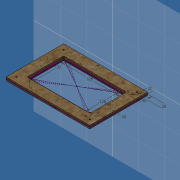
# Autodesk Inventor part: Flachfilter_Rahmen
Saved by Autodesk Inventor 2019 (Build 230136000, 136)
## iProperties
Created: 2020-08-04
Part Number: Flachfilter_Rahmen
Material: Generisch
Document SubType Name: Modeling
Designer: Stefan
Mass: 458.465 g
Surface Area: 1020.14 cm^2
Volume: 458.465 cm^3
Density: 1 g/cm^3
Appearance: Spanplatte
Author: Stefan
Autodesk Inventor part; units mm, degrees
ref_plane "YZ Plane" through (0, 0, 0) normal (1, 0, 0) x (0, 1, 0)
ref_plane "XZ Plane" through (0, 0, 0) normal (0, 1, 0) x (-1, 0, 0)
ref_plane "XY Plane" through (0, 0, 0) normal (0, 0, 1) x (1, 0, 0)
sketch "Skizze1" plane through (0, 0, 0) normal (0, 1, 0) x (-1, 0, 0)
  arc A0 (-116, -64) -> (-114, -66) centre (-114, -64) ccw
  arc A1 (-114, -62) -> (-112, -64) centre (-112, -62) ccw
  line L0 (-114, -62) -> (-114, 62)
  line L1 (-116, 64) -> (-116, -64)
  line L2 (-120, -65) -> (-120, 65)
  line L3 (112, -64) -> (-112, -64)
  line L4 (-114, -66) -> (114, -66)
  line L5 (115, -70) -> (-115, -70)
  line L6 (-112, 64) -> (112, 64)
  line L7 (114, 64) -> (-114, -64) construction
  line L8 (114, 66) -> (-114, 66)
  line L9 (-116, 66) -> (116, -66) construction
  line L10 (-116, -66) -> (116, 66) construction
  line L11 (-115, 70) -> (115, 70)
  line L12 (120, 70) -> (-120, -70) construction
  line L13 (120, -70) -> (-120, 70) construction
  line L14 (114, -64) -> (-114, 64) construction
  line L15 (120, 65) -> (120, -65)
  arc A2 (-120, -65) -> (-115, -70) centre (-115, -65) ccw
  arc A3 (-112, 64) -> (-114, 62) centre (-112, 62) ccw
  arc A4 (-115, 70) -> (-120, 65) centre (-115, 65) ccw
  arc A5 (-114, 66) -> (-116, 64) centre (-114, 64) ccw
  arc A6 (120, 65) -> (115, 70) centre (115, 65) ccw
  arc A7 (115, -70) -> (120, -65) centre (115, -65) ccw
  line L16 (116, -64) -> (116, 64)
  arc A8 (114, -66) -> (116, -64) centre (114, -64) ccw
  arc A9 (112, -64) -> (114, -62) centre (112, -62) ccw
  line L17 (114, 62) -> (114, -62)
  arc A10 (114, 62) -> (112, 64) centre (112, 62) ccw
  arc A11 (116, 64) -> (114, 66) centre (114, 64) ccw
  line L18 (-160, -110) -> (160, -110)
  line L19 (160, -110) -> (160, 110)
  line L20 (160, 110) -> (-160, 110)
  line L21 (-160, 110) -> (-160, -110)
  line L22 (-160, -110) -> (160, 110) construction
  line L23 (160, -110) -> (-160, 110) construction
  circle A12 centre (-140, -90) radius 2.75
  line L24 (140, 90) -> (-140, 90)
  line L25 (-140, 90) -> (-140, -90)
  line L26 (-140, -90) -> (140, -90)
  line L27 (140, -90) -> (140, 90)
  line L28 (140, 90) -> (-140, -90) construction
  line L29 (-140, 90) -> (140, -90) construction
  circle A13 centre (140, -90) radius 2.75
  circle A14 centre (140, 90) radius 2.75
  circle A15 centre (-140, 90) radius 2.75
  point P0 (0, 0)
  point P1 (0, 0)
  point P2 (0, 0)
  point P3 (0, 0)
  point P4 (0, 0)
  point P5 (0, 0)
  point P6 (0, 0)
  dimension "d0" = 140
  dimension "d1" = 240
  dimension "d2" = 5
  dimension "d3" = 232
  dimension "d4" = 132
  dimension "d5" = 2
  dimension "d6" = 128
  dimension "d7" = 228
  dimension "d8" = 2
  dimension "d19" = 40
  dimension "d20" = 40
  dimension "d21" = 5.5
  dimension "d23" = 20
  dimension "d24" = 20
  constraints: 60 end point, 24 point on circle, 24 point on line, 24 tangent, 16 centre point, 15 midpoint, 12 equal radius, 12 parallel, 5 coincident, 5 perpendicular, 3 horizontal
  measures "d0" distance of L12.end L13.end
  measures "d1" distance of L13.start L12.end
  measures "d2" radius of A6
  measures "d3" distance of L10.start L9.end
  measures "d4" distance of L9.end L10.end
  measures "d5" radius of A8
  measures "d6" distance of L7.end L14.end
  measures "d7" distance of L14.start L7.end
  measures "d8" radius of A9
  measures "d19" distance between parallel lines of L5 L18
  measures "d20" distance between parallel lines of L2 L21
  measures "d21" diameter of A12
  measures "d23" distance between parallel lines of L18 L26
  measures "d24" distance between parallel lines of L25 L21
extrude "Extrusion1" add sketch "Skizze1" along normal blind 6 contours L21 L20 L19 L18 | L26 L25 A12 | A12 L25 L26 | A12 L25 A15 L24 A14 L27 A13 L26 | A13 L27 L26 | L26 L27 A13 | A15 L24 L25 | L25 L24 A15 | A14 L24 L27 | L27 L24 A14
extrude "Extrusion2" add sketch "Skizze1" against normal blind 6 contours L2 A4 L11 A6 L15 A7 L5 A2 | L21 L20 L19 L18 | L26 L25 A12 | A12 L25 L26 | A12 L25 A15 L24 A14 L27 A13 L26 | A13 L27 L26 | L26 L27 A13 | A15 L24 L25 | L25 L24 A15 | A14 L24 L27 | L27 L24 A14
extrude "Extrusion3" cut sketch "Skizze1" along normal through all both and the other way through all contours L26 L25 A12 | A12 L25 L26 | A13 L27 L26 | L26 L27 A13 | A15 L24 L25 | L25 L24 A15 | A14 L24 L27 | L27 L24 A14
equation "\"d14\" = mdf_thickness"
equation "\"d16\" = mdf_thickness"
equation "\"d10\" = 6"
equation "\"kg_thickness\" = 4.9"
equation "\"ht_thickness\" = 1.9"
equation "\"case_thickness\" = 18"
equation "\"inner_thickness\" = 15"
equation "\"gap_fit\" = 0.1"
equation "\"gap_slide\" = 0.2"
equation "\"gap_air\" = 1"
equation "\"bore_diameter\" = 73"
equation "\"mdf_thickness\" = 6"
equation "\"tape_width\" = 15"
equation "\"tape_thickness\" = 3"
equation "\"inner_depth\" = 255"
